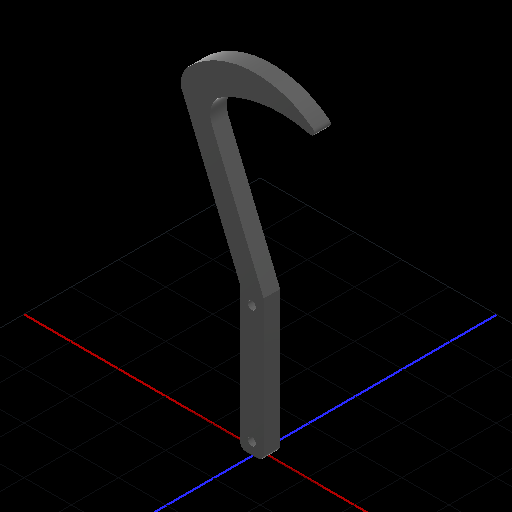
# Autodesk Inventor part: wing
Saved by Autodesk Inventor 2025.2 (Build 292293000, 293)
## iProperties
Created: 2026-01-05
Part Number: wing
Material: Acetal Resin, Black
Document SubType Name: Modeling
Designer: cloudy
Density: 1.425 g/cm^3
Appearance: Smooth - Black
Author: cloudy
Autodesk Inventor part; units mm, degrees
ref_plane "YZ Plane" through (0, 0, 0) normal (1, 0, 0) x (0, 1, 0)
ref_plane "XY Plane" through (0, 0, 0) normal (0, 0, 1) x (1, 0, 0)
sketch "Sketch1" plane through (0, 0, 0) normal (0, 1, 0) x (-1, 0, 0)
  line L0 (6.35, 4.445) -> (-6.35, 4.445)
  line L1 (-6.35, 4.445) -> (-6.35, -4.445)
  line L2 (-6.35, -4.445) -> (6.35, -4.445)
  line L3 (6.35, -4.445) -> (6.35, 4.445)
  line L4 (6.35, 4.445) -> (-6.35, -4.445) construction
  line L5 (-6.35, 4.445) -> (6.35, -4.445) construction
  line L6 (0, 0) -> (0, -5.5773) construction
  dimension "d0" = 90
  dimension "d1" = 12.7
  dimension "d2" = 8.89
  constraints: 14 end point, 2 midpoint, 2 parallel, 1 perpendicular, 1 vertical
  measures "d0" angle of L0 L6
  measures "d1" distance of L0.start L0.end
  measures "d2" distance of L2.end L0.start
ref_plane "Work Plane1" through (0, 152.4, 0) normal (0, 1, 0) x (-1, 0, 0)
sketch "Sketch2" plane through (0, 152.4, 0) normal (0, 1, 0) x (-1, 0, 0)
  line L0 (38.1, 4.445) -> (25.4, 4.445)
  line L1 (25.4, 4.445) -> (25.4, -4.445)
  line L2 (25.4, -4.445) -> (38.1, -4.445)
  line L3 (38.1, -4.445) -> (38.1, 4.445)
  line L4 (38.1, 4.445) -> (25.4, -4.445) construction
  line L5 (25.4, 4.445) -> (38.1, -4.445) construction
  line L6 (0, 0) -> (31.75, 0) construction
  dimension "d4" = 8.89
  dimension "d5" = 12.7
  dimension "d25" = 31.75
  constraints: 14 end point, 2 horizontal, 2 midpoint, 2 parallel, 1 perpendicular
  measures "d4" distance of L2.end L0.start
  measures "d5" distance of L0.start L0.end
  measures "d25" distance of L6.start L6.end
extrude "Extrusion1" add sketch "Sketch1" along normal blind 76.2
loft "Loft1" add profiles "Sketch2" section 1 edges at (6.35, 76.2, 0) (0, 76.2, -4.445) (-6.35, 76.2, 0) (0, 76.2, 4.445)
ref_plane "Work Plane2" through (-31.75, 152.4, 4.445) normal (0, 0, 1) x (1, 0, 0)
sketch "Sketch3" plane through (-31.75, 152.4, 4.445) normal (0, 0, 1) x (1, 0, 0)
  line L0 (25.4, -76.2) -> (-6.35, 0) projected
  line L1 (38.1, -76.2) -> (6.35, 0) projected
  line L2 (-6.35, 0) -> (6.35, 0)
  arc A0 (71.2588, 9.8335) -> (6.35, 0) centre (46.9465, -48.828) ccw
  arc A1 (71.2588, 9.8335) -> (-6.35, 7.1942) centre (33.5678, -24.2257) ccw
  line L3 (-6.35, 7.1942) -> (-6.35, 0)
  point P0 (31.75, -152.4)
  dimension "d12" = 50.8
  dimension "d13" = 63.5
  constraints: 4 end point, 4 point on circle, 2 centre point, 1 horizontal, 1 vertical
  measures "d12" radius of A1
  measures "d13" radius of A0
extrude "Extrusion2" add sketch "Sketch3" against normal up to surface (8.89 mm away)
sketch "Sketch4" plane through (6.35, 0, 4.445) normal (0, 0, 1) x (1, 0, 0)
  circle A0 centre (-6.35, 6.35) radius 2.1844
  circle A1 centre (-6.35, 69.85) radius 2.1844
  line L0 (-6.35, 0) -> (-6.35, 69.85) construction
  line L1 (-12.7, 0) -> (0, 0) construction
  dimension "d16" = 4.3688
  dimension "d17" = 4.3688
  dimension "d18" = 63.5
  dimension "d19" = 6.35
  constraints: 2 centre point, 2 end point, 1 point on line, 1 vertical
  measures "d16" diameter of A0
  measures "d17" diameter of A1
  measures "d18" distance of L0.end A0.centre
  measures "d19" distance from line of L1 A0.centre
extrude "Extrusion3" cut sketch "Sketch4" against normal through all
fillet "Fillet1" radius 3.175 2 edges at (-6.35, 0, 0) (6.35, 0, 0)
fillet "Fillet2" radius 1.905 1 edges at (39.5088, 162.2335, 0)
fillet "Fillet3" radius 12.7 2 edges at (-38.1, 159.5942, 0) (-25.4, 152.4, 0)
body "Solid1"
